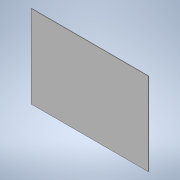
# Autodesk Inventor part: A4 ref plane
Saved by Autodesk Inventor 2021 (Build 250183000, 183)
## iProperties
Created: 2023-10-27
Part Number: A4 ref plane
Material: Generic
Document SubType Name: Modeling
Designer: Toby
Density: 1 g/cm^3
Appearance: Default
Author: Toby
Autodesk Inventor part; units mm, degrees
ref_plane "YZ Plane" through (0, 0, 0) normal (1, 0, 0) x (0, 1, 0)
ref_plane "XZ Plane" through (0, 0, 0) normal (0, 1, 0) x (-1, 0, 0)
ref_plane "XY Plane" through (0, 0, 0) normal (0, 0, 1) x (1, 0, 0)
sketch "Sketch1" plane through (0, 0, 0) normal (0, 0, 1) x (1, 0, 0)
  line L0 (-262.8777, 110.0989) -> (34.1223, 110.0989)
  line L1 (34.1223, 110.0989) -> (34.1223, -99.9011)
  line L2 (34.1223, -99.9011) -> (-262.8777, -99.9011)
  line L3 (-262.8777, -99.9011) -> (-262.8777, 110.0989)
  point P0 (0, 0)
  dimension "d0" = 210
  dimension "d1" = 297
  constraints: 8 end point, 2 parallel, 1 horizontal, 1 perpendicular
  measures "d0" distance of L2.end L0.start
  measures "d1" distance of L0.start L0.end
extrude "Extrusion1" add sketch "Sketch1" along normal blind 1
body "Solid1"
